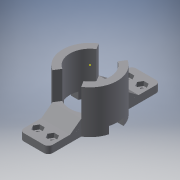
# Autodesk Inventor part: SuporteMotor
Saved by Autodesk Inventor 2019.4 (Build 234330000, 330)
## iProperties
Created: 2019-10-16
Part Number: SuporteMotor
Material: Genérico
Document SubType Name: Modeling
Designer: natha
Density: 1 g/cm^3
Appearance: Padrão
Author: natha
Autodesk Inventor part; units mm, degrees
ref_plane "YZ Plane" through (0, 0, 0) normal (1, 0, 0) x (0, 1, 0)
sketch "Esboço1" plane through (0, 0, 0) normal (0, 1, 0) x (-1, 0, 0)
  circle A0 centre (0, 0) radius 19
  circle A1 centre (0, 0) radius 14
  dimension "d0" = 38
  dimension "d1" = 28
  constraints: 2 centre point, 2 coincident
  measures "d0" diameter of A0
  measures "d1" diameter of A1
extrude "Extrusão1" add sketch "Esboço1" along normal blind 30
sketch "Esboço2" plane through (0, 0, 0) normal (1, 0, 0) x (0, 1, 0)
  line L0 (-5, 5) -> (5, 5)
  line L1 (5, 5) -> (5, -5)
  line L2 (5, -5) -> (-5, -5)
  line L3 (-5, -5) -> (-5, 5)
  line L4 (-5, 5) -> (5, -5) construction
  line L5 (5, 5) -> (-5, -5) construction
  point P0 (0, 0)
  dimension "d4" = 10
  dimension "d5" = 10
  constraints: 12 end point, 2 midpoint, 2 parallel, 1 horizontal, 1 perpendicular
  measures "d4" distance of L1.end L2.end
  measures "d5" distance of L2.end L0.start
extrude "Extrusão2" cut sketch "Esboço2" along normal mid plane 40
sketch "Esboço3" plane through (0, 0, 0) normal (0, 0, 1) x (1, 0, 0)
  point P0 (0, 0)
ref_plane "Plano de trabalho1" through (0, 30, 0) normal (0, 1, 0) x (-1, 0, 0)
sketch "Esboço4" plane through (0, 30, 0) normal (0, 1, 0) x (-1, 0, 0)
  circle A0 centre (0, 0) radius 19 projected
  line L0 (10.0122, 16.148) -> (-10.0122, -16.148) construction
  line L1 (-10.0122, 16.148) -> (10.0122, -16.148) construction
  circle A1 centre (0, 0) radius 14 projected
  line L2 (7.3774, 11.8985) -> (-7.3774, -11.8985) construction
  line L3 (-7.3774, 11.8985) -> (7.3774, -11.8985) construction
  line L4 (10.0122, -16.148) -> (7.3774, -11.8985)
  line L5 (-10.0122, -16.148) -> (-7.3774, -11.8985)
  line L6 (-10.0122, 16.148) -> (-7.3774, 11.8985)
  line L7 (7.3774, 11.8985) -> (10.0122, 16.148)
  arc A2 (-10.0122, -16.148) -> (10.0122, -16.148) centre (0, 0) ccw
  arc A3 (10.0122, 16.148) -> (-10.0122, 16.148) centre (0, 0) ccw
  arc A4 (7.3774, 11.8985) -> (-7.3774, 11.8985) centre (0, 0) ccw
  arc A5 (-7.3774, -11.8985) -> (7.3774, -11.8985) centre (0, 0) ccw
  constraints: 17 end point, 11 point on circle, 4 centre point, 4 midpoint, 3 point on line, 2 coincident
extrude "Extrusão3" cut sketch "Esboço4" against normal blind 19.3 contours L7 A1 L6 A0 | A0 L5 A1 L4
sketch "Esboço5" plane through (0, 30, 0) normal (0, 1, 0) x (-1, 0, 0)
  point P0 (0, 0)
ref_plane "Plano de trabalho4" through (0, 0, 19) normal (0, 0, 1) x (1, 0, 0)
sketch "Esboço6" plane through (0, 0, 19) normal (0, 0, 1) x (1, 0, 0)
  line L0 (-10.0122, 10.7) -> (-7.3774, 10.7) projected
  line L1 (7.3774, 10.7) -> (10.0122, 10.7) projected
  line L2 (13.0767, 0) -> (-13.0767, 0) projected
  line L3 (10.0122, 0) -> (-10.0122, 0)
  line L4 (-10.0122, 0) -> (10.0122, 0)
  line L5 (10.0122, 0) -> (10.0122, 5)
  line L6 (10.0122, 5) -> (-10.0122, 5)
  line L7 (-10.0122, 5) -> (-10.0122, 0)
  point P0 (0, 0)
  dimension "d20" = 5
  constraints: 10 end point, 2 parallel, 1 collinear, 1 horizontal, 1 perpendicular, 1 point on line
  measures "d20" distance of L4.end L5.end
extrude "Extrusão4" add sketch "Esboço6" along normal blind 20.048 and the other way blind 3
fillet "Arredondamento1" radius 3 2 edges at (-10.0122, 2.5, 39.048) (10.0122, 2.5, 39.048)
sketch "Esboço7" plane through (0, 0, 0) normal (1, 0, 0) x (0, 1, 0)
  line L0 (10.7, 16.148) -> (10.7, 11.8985) projected
  line L1 (5, 36.048) -> (5, 16.148) projected
  line L2 (10.7, 16.148) -> (5, 16.148)
  line L3 (5, 16.148) -> (5, 23.848)
  line L4 (5, 23.848) -> (10.7, 23.848)
  line L5 (10.7, 23.848) -> (10.7, 16.148)
  point P0 (0, 0)
  dimension "d28" = 7.7
  constraints: 8 end point, 2 parallel, 1 horizontal, 1 perpendicular, 1 point on line
  measures "d28" distance of L4.end L0.start
extrude "Extrusão5" add sketch "Esboço7" along normal mid plane 20
chamfer "Chanfro1" distance 5.7 distance2 7.7 1 edges at (0, 10.7, 23.848) measured on face at (-3.3333, 6.9, 23.848)
sketch "Esboço8" plane through (-7.0122, 5, 39.048) normal (0, 1, 0) x (1, 0, 0)
  line L0 (0, 0) -> (14.0243, 0) projected
  line L1 (1.9995, 0) -> (1.9995, 7.85) construction
  line L2 (5.3995, 7.85) -> (3.6995, 4.9055)
  line L3 (3.6995, 4.9055) -> (0.2995, 4.9055)
  line L4 (0.2995, 4.9055) -> (-1.4005, 7.85)
  line L5 (-1.4005, 7.85) -> (0.2995, 10.7945)
  line L6 (0.2995, 10.7945) -> (3.6995, 10.7945)
  line L7 (3.6995, 10.7945) -> (5.3995, 7.85)
  line L8 (5.3995, 7.85) -> (8.5995, 7.85) construction
  line L9 (11.9995, 0) -> (11.9995, 7.85) construction
  line L10 (15.3995, 7.85) -> (13.6995, 4.9055)
  line L11 (13.6995, 4.9055) -> (10.2995, 4.9055)
  line L12 (10.2995, 4.9055) -> (8.5995, 7.85)
  line L13 (8.5995, 7.85) -> (10.2995, 10.7945)
  line L14 (10.2995, 10.7945) -> (13.6995, 10.7945)
  line L15 (13.6995, 10.7945) -> (15.3995, 7.85)
  line L16 (-1.4005, 7.85) -> (-3.0005, 7.85) construction
  line L17 (15.3995, 7.85) -> (16.9995, 7.85) construction
  line L18 (17.0243, 3) -> (17.0243, 22.9) projected
  line L19 (-3, 3) -> (-3, 22.9) projected
  line L20 (-3, 22.9) -> (-3, 3) projected
  point P0 (7.0122, 39.048)
  point P1 (-3, 7.85)
  dimension "d37" = 7.85
  dimension "d38" = 3.4
  dimension "d39" = 3.2
  dimension "d40" = 7.85
  dimension "d41" = 3.4
  dimension "d43" = 16.8
  dimension "d44" = 1.6
  dimension "d45" = 1.6
  constraints: 34 end point, 3 horizontal, 2 coincident, 2 vertical, 1 point on line, 26 other
  measures "d37" distance of L1.start L1.end
  measures "d38" distance of L5.end L6.end
  measures "d39" distance of L2.start L8.end
  measures "d40" distance of L9.start L9.end
  measures "d41" distance of L13.end L14.end
  measures "d43" distance of L10.start L4.end
  measures "d44" distance of L4.end L16.end
  measures "d45" distance of L10.start L17.end
ref_plane "Plano de trabalho5" through (0, 0, 16.148) normal (0, 0, 1) x (1, 0, 0)
extrude "Extrusão6" cut sketch "Esboço8" against normal blind 3
sketch "Esboço9" plane through (-7.0122, 2, 39.048) normal (0, 1, 0) x (1, 0, 0)
  line L0 (0.2995, 10.7945) -> (3.6995, 10.7945) construction
  line L1 (5.3995, 7.85) -> (3.6995, 4.9055) projected
  line L2 (3.6995, 10.7945) -> (5.3995, 7.85) projected
  line L3 (0.2995, 10.7945) -> (3.6995, 10.7945) projected
  line L4 (-1.4005, 7.85) -> (0.2995, 10.7945) projected
  line L5 (0.2995, 4.9055) -> (-1.4005, 7.85) projected
  line L6 (3.6995, 4.9055) -> (0.2995, 4.9055) projected
  line L7 (3.6995, 10.7945) -> (0.2995, 4.9055) construction
  line L8 (0.2995, 10.7945) -> (3.6995, 4.9055) construction
  circle A0 centre (1.9995, 7.85) radius 1.8
  line L9 (15.3995, 7.85) -> (13.6995, 4.9055) construction
  line L10 (13.6995, 10.7945) -> (15.3995, 7.85) construction
  line L11 (10.2995, 10.7945) -> (13.6995, 10.7945) construction
  line L12 (8.5995, 7.85) -> (10.2995, 10.7945) construction
  line L13 (10.2995, 4.9055) -> (8.5995, 7.85) construction
  line L14 (13.6995, 4.9055) -> (10.2995, 4.9055) construction
  line L15 (13.6995, 10.7945) -> (10.2995, 4.9055) construction
  line L16 (10.2995, 10.7945) -> (13.6995, 4.9055) construction
  circle A1 centre (11.9995, 7.85) radius 1.8
  point P0 (7.0122, 39.048)
  dimension "d49" = 3.6
  dimension "d50" = 3.6
  constraints: 8 end point, 2 centre point, 2 midpoint
  measures "d49" diameter of A0
  measures "d50" diameter of A1
extrude "Extrusão7" cut sketch "Esboço9" against normal up to next contours A0 | A1
mirror "Espelhamento1" about plane through (0, 0, 0) normal (0, 0, 1) of "Extrusão4", "Arredondamento1", "Extrusão5", "Chanfro1", "Extrusão6", "Extrusão7"
sketch "Esboço11" plane through (-10, 5, -16.1555) normal (-1, 0, 0) x (0, 0, 1)
  line L0 (0, 5.6944) -> (-7.6925, 0) projected
  line L1 (0, 5.7) -> (-7.6925, 5.7)
  line L2 (-7.6925, 5.7) -> (-7.6925, 0)
  line L3 (-7.6925, 0) -> (0, 5.7)
  point P0 (16.1555, -5)
  point P1 (0, 0)
  constraints: 6 end point
extrude "Extrusão9" cut sketch "Esboço11" against normal blind 20
sketch "Esboço12" plane through (0, 0, 0) normal (0, -1, 0) x (1, 0, 0)
  circle A0 centre (-5.0126, 31.198) radius 1.8 projected
  circle A1 centre (4.9874, 31.198) radius 1.8 projected
  circle A2 centre (4.9874, -31.198) radius 1.8 projected
  circle A3 centre (-5.0126, -31.198) radius 1.8 projected
  point P0 (0, 0)
